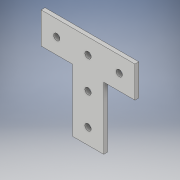
# Autodesk Inventor part: T-Gusset
Saved by Autodesk Inventor 2018 (Build 220112000, 112)
## iProperties
Created: 2020-05-06
Part Number: T-Gusset
Material: Generic
Document SubType Name: Modeling
Designer: maste
Density: 1 g/cm^3
Appearance: Default
Author: maste
Autodesk Inventor part; units mm, degrees
ref_plane "YZ Plane" through (0, 0, 0) normal (1, 0, 0) x (0, 1, 0)
ref_plane "XZ Plane" through (0, 0, 0) normal (0, 1, 0) x (-1, 0, 0)
ref_plane "XY Plane" through (0, 0, 0) normal (0, 0, 1) x (1, 0, 0)
sketch "Sketch1" plane through (0, 0, 0) normal (0, 0, 1) x (1, 0, 0)
  line L0 (76.2, 0) -> (76.2, 25.4)
  line L1 (76.2, 25.4) -> (0, 25.4)
  line L2 (0, 25.4) -> (0, 0)
  line L3 (0, 0) -> (25.4, 0) construction
  line L4 (25.4, 0) -> (25.4, -50.8)
  line L5 (25.4, -50.8) -> (50.8, -50.8)
  line L6 (50.8, -50.8) -> (50.8, 0)
  line L7 (0, 0) -> (25.4, 0)
  line L8 (50.8, 0) -> (76.2, 0)
  line L9 (0, 12.7) -> (12.7, 12.7) construction
  line L10 (12.7, 12.7) -> (38.1, 12.7) construction
  line L11 (38.1, 12.7) -> (63.5, 12.7) construction
  line L12 (38.1, 12.7) -> (38.1, -12.7) construction
  line L13 (38.1, -12.7) -> (38.1, -38.1) construction
  circle A0 centre (12.7, 12.7) radius 2.5781
  circle A1 centre (38.1, 12.7) radius 2.5781
  circle A2 centre (63.5, 12.7) radius 2.5781
  circle A3 centre (38.1, -12.7) radius 2.5781
  circle A4 centre (38.1, -38.1) radius 2.5781
  dimension "d0" = 76.2
  dimension "d1" = 25.4
  dimension "d2" = 25.4
  dimension "d3" = 50.8
  dimension "d4" = 25.4
  dimension "d5" = 25.4
  dimension "d6" = 25.4
  dimension "d7" = 5.1562
  constraints: 28 end point, 6 perpendicular, 5 centre point, 5 coincident, 3 horizontal, 3 parallel, 3 point on line, 1 midpoint, 1 vertical
  measures "d0" distance of L1.end L0.end
  measures "d1" distance of L0.end L0.start
  measures "d2" distance of L2.end L3.end
  measures "d3" distance of L3.end L4.end
  measures "d4" distance of L4.end L5.end
  measures "d5" distance of L10.end L12.end
  measures "d6" distance of L12.end L13.end
  measures "d7" diameter of A0
extrude "Extrusion1" add sketch "Sketch1" along normal blind 3.175
body "Solid1"
